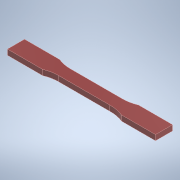
# Autodesk Inventor part: TensileTestSpecimen
Saved by Autodesk Inventor 2022 (Build 260153000, 153)
## iProperties
Created: 2021-11-02
Part Number: TensileTestSpecimen
Material: Genérico
Document SubType Name: Modeling
Designer: JK
Density: 1 g/cm^3
Appearance: Castaño
Author: JK
Autodesk Inventor part; units mm, degrees
ref_plane "YZ Plane" through (0, 0, 0) normal (1, 0, 0) x (0, 1, 0)
ref_plane "XZ Plane" through (0, 0, 0) normal (0, 1, 0) x (-1, 0, 0)
ref_plane "XY Plane" through (0, 0, 0) normal (0, 0, 1) x (1, 0, 0)
sketch "Boceto1" plane through (0, 0, 0) normal (0, 1, 0) x (-1, 0, 0)
  line L0 (-28.5, 6.5) -> (28.5, 6.5)
  line L1 (28.5, 6.5) -> (28.5, -6.5)
  line L2 (28.5, -6.5) -> (-28.5, -6.5)
  line L3 (-28.5, -6.5) -> (-28.5, 6.5)
  line L4 (-28.5, 6.5) -> (28.5, -6.5) construction
  line L5 (28.5, 6.5) -> (-28.5, -6.5) construction
  line L6 (82.5, 9.5) -> (28.5, 9.5)
  line L7 (28.5, 9.5) -> (28.5, -9.5)
  line L8 (28.5, -9.5) -> (82.5, -9.5)
  line L9 (82.5, -9.5) -> (82.5, 9.5)
  line L10 (-28.5, 9.5) -> (-82.5, 9.5)
  line L11 (-82.5, 9.5) -> (-82.5, -9.5)
  line L12 (-82.5, -9.5) -> (-28.5, -9.5)
  line L13 (-28.5, -9.5) -> (-28.5, 9.5)
  point P0 (0, 0)
  point P1 (28.5, 6.5)
  point P2 (-28.5, 6.5)
  point P3 (28.5, -6.5)
  dimension "d0" = 13
  dimension "d1" = 57
  dimension "d2" = 19
  dimension "d3" = 9.5
  dimension "d4" = 9.5
  dimension "d5" = 19
  dimension "d6" = 165
  constraints: 28 end point, 6 parallel, 3 collinear, 3 horizontal, 3 perpendicular, 2 midpoint
  measures "d0" distance between parallel lines of L2 L0
  measures "d1" distance of L1.end L2.end
  measures "d2" distance of L8.end L6.start
  measures "d3" distance from line of point (0, 0) L6
  measures "d4" distance from line of point (0, 0) L10
  measures "d5" distance of L10.end L11.end
  measures "d6" distance between parallel lines of L9 L11
extrude "Extrusión1" add sketch "Boceto1" along normal mid plane 6
sketch "Boceto3" plane through (0, 3, 0) normal (0, 1, 0) x (1, 0, 0)
  circle A0 centre (-28.5074, -44.5) radius 38
  line L0 (-28.5, -6.5) -> (28.5, -6.5) projected
  circle A1 centre (-28.5074, 44.5) radius 38
  circle A2 centre (29.8049, 44.5) radius 38
  circle A3 centre (29.8049, -44.5) radius 38
  line L1 (28.5, 6.5) -> (-28.5, 6.5) projected
  point P0 (0, 0)
  point P1 (0.6488, -68.8704)
  point P2 (0.6488, -20.1296)
  point P3 (0.6488, 68.8704)
  point P4 (0.6488, 20.1296)
  dimension "d11" = 76
  constraints: 4 centre point, 3 equal radius, 2 horizontal alignment, 2 tangent, 2 vertical alignment
  measures "d11" diameter of A0
extrude "Extrusión2" cut sketch "Boceto3" against normal through all
